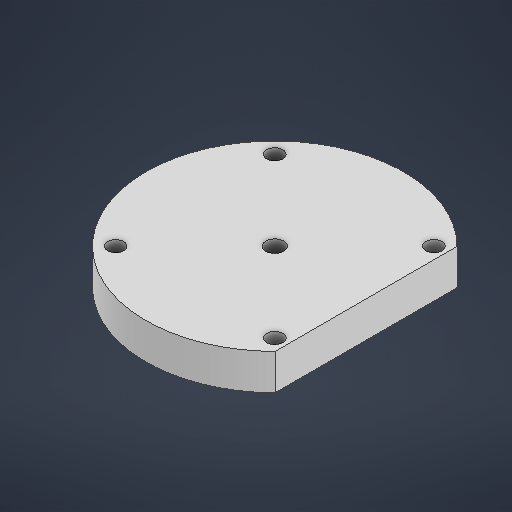
# Autodesk Inventor part: Bottom Cap outlet
Saved by Autodesk Inventor 2025 (Build 290162000, 162)
## iProperties
Created: 2024-07-01
Part Number: Bottom Cap outlet
Material: Generic
Document SubType Name: Modeling
Designer: mayhe
Density: 1 g/cm^3
Appearance: Default
Author: mayhe
Autodesk Inventor part; units mm, degrees
ref_plane "YZ Plane" through (0, 0, 0) normal (1, 0, 0) x (0, 1, 0)
ref_plane "XZ Plane" through (0, 0, 0) normal (0, 1, 0) x (-1, 0, 0)
ref_plane "XY Plane" through (0, 0, 0) normal (0, 0, 1) x (1, 0, 0)
sketch "Sketch1" plane through (0, 0, 0) normal (0, 1, 0) x (-1, 0, 0)
  circle A0 centre (0, 0) radius 36
  line L0 (-22.225, 22.225) -> (22.225, 22.225)
  line L1 (22.225, 22.225) -> (22.225, -22.225)
  line L2 (22.225, -22.225) -> (-22.225, -22.225)
  line L3 (-22.225, -22.225) -> (-22.225, 22.225)
  line L4 (-22.225, 22.225) -> (22.225, -22.225) construction
  line L5 (22.225, 22.225) -> (-22.225, -22.225) construction
  circle A1 centre (0, 0) radius 32.5
  circle A2 centre (22.225, -22.225) radius 2.25
  circle A3 centre (22.225, 22.225) radius 2.25
  circle A4 centre (-22.225, 22.225) radius 2.25
  circle A5 centre (-22.225, -22.225) radius 2.25
  line L6 (-25.512, 25.3996) -> (-25.512, -25.3996)
  dimension "d0" = 72
  dimension "d1" = 44.45
  dimension "d2" = 44.45
  dimension "d3" = 65
  dimension "d4" = 4.5
  dimension "d5" = 4.5
  dimension "d6" = 4.5
  dimension "d7" = 4.5
  dimension "d9" = 25.512
  dimension "d10" = 3.287
  constraints: 14 end point, 6 centre point, 6 coincident, 2 midpoint, 2 parallel, 2 point on circle, 1 horizontal, 1 perpendicular, 1 vertical
  measures "d0" diameter of A0
  measures "d1" distance of L1.end L2.end
  measures "d2" distance of L0.end L1.end
  measures "d3" diameter of A1
  measures "d4" diameter of A2
  measures "d5" diameter of A3
  measures "d6" diameter of A4
  measures "d7" diameter of A5
  measures "d9" distance from line of L6 A0.centre
  measures "d10" distance between parallel lines of L6 L3
extrude "Extrusion1" add sketch "Sketch1" along normal blind 10 contours A0 L6 A1 A5 A2 A3 A4 | A1 A4 L3 A5 L6 | A1 A3 L0 A4 | A4 L0 A3 L1 A2 L2 A5 L3 | A5 L2 A2 A1 | A1 A2 L1 A3
sketch "Sketch2" plane through (0, 10, 0) normal (0, 1, 0) x (1, 0, 0)
  circle A0 centre (0, 0) radius 2.5
  dimension "d13" = 5
  constraints: 1 centre point, 1 coincident
  measures "d13" diameter of A0
extrude "Extrusion2" cut sketch "Sketch2" against normal blind 10
body "Solid1"
